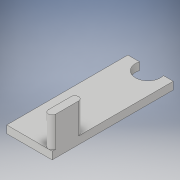
# Autodesk Inventor part: piston locking tool
Saved by Autodesk Inventor 2018 (Build 220112000, 112)
## iProperties
Created: 2019-03-02
Part Number: piston locking tool
Material: Generic
Document SubType Name: Modeling
Designer: s-4008082
Density: 1 g/cm^3
Appearance: Default
Author: s-4008082
Autodesk Inventor part; units mm, degrees
ref_plane "YZ Plane" through (0, 0, 0) normal (1, 0, 0) x (0, 1, 0)
ref_plane "XZ Plane" through (0, 0, 0) normal (0, 1, 0) x (-1, 0, 0)
ref_plane "XY Plane" through (0, 0, 0) normal (0, 0, 1) x (1, 0, 0)
sketch "Sketch1" plane through (0, 0, 0) normal (0, 1, 0) x (-1, 0, 0)
  line L0 (0, 0) -> (-19.05, 0)
  line L1 (-19.05, 0) -> (-19.05, 50.8)
  line L2 (-19.05, 50.8) -> (0, 50.8)
  line L3 (0, 50.8) -> (0, 0)
  circle A0 centre (-9.525, 3.175) radius 6.35
  point P0 (-1.5875, 0)
  point P1 (-11.1125, 0)
  dimension "d1" = 19.05
  dimension "d4" = 50.8
  dimension "d11" = 12.7
  dimension "d12" = 3.175
  dimension "d13" = 9.525
  constraints: 8 end point, 2 parallel, 2 point on line, 1 centre point, 1 horizontal, 1 perpendicular
  measures "d1" distance between parallel lines of L3 L1
  measures "d4" distance of L2.end L0.start
  measures "d11" diameter of A0
  measures "d12" distance from line of L0 A0.centre
  measures "d13" distance from line of L1 A0.centre
extrude "Extrusion1" add sketch "Sketch1" along normal blind 3.175 contours L0 A0 L1 L2 L3 | L0 A0 picked at (-8.7548, 5.6041)
sketch "Sketch2" plane through (0, 3.175, 0) normal (0, 1, 0) x (1, 0, 0)
  line L0 (17.4625, -49.2125) -> (17.4625, -39.6875) construction
  line L1 (19.05, -49.2125) -> (19.05, -39.6875)
  line L2 (15.875, -39.6875) -> (15.875, -49.2125)
  arc A0 (15.875, -49.2125) -> (19.05, -49.2125) centre (17.4625, -49.2125) ccw
  arc A1 (19.05, -39.6875) -> (15.875, -39.6875) centre (17.4625, -39.6875) ccw
  line L3 (0, -50.8) -> (19.05, -50.8) projected
  line L4 (19.05, -50.8) -> (19.05, 0) projected
  point P0 (0, 0)
  point P1 (17.4625, -44.45)
  dimension "d23" = 1.5875
  dimension "d24" = 1.5875
  dimension "d25" = 9.525
  dimension "d26" = 0
  constraints: 8 end point, 4 point on circle, 4 tangent, 2 centre point, 1 midpoint, 1 parallel
  measures "d23" distance from line of L3 L0.start
  measures "d24" distance from line of L0.start L1
  measures "d25" distance of L2.start L2.end
  measures "d26" distance between parallel lines of L4 L1
extrude "Extrusion2" add sketch "Sketch2" along normal blind 12.7 contours A0 L2 A1 L1
hole "Hole1" at (9.9145, 3.175, 1.4669) direction (0, -1, 0) diameter 10.4588 end through all
body "Solid1"
